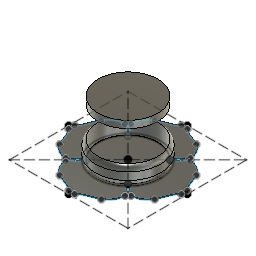
base (Autodesk Fusion 360 design; units mm, degrees)
Autodesk Fusion 360 part; units mm, degrees
note: some values were not read from the file. Set by a fixed rule: which sketch regions a step uses.
sketch "Sketch1" plane through (0, 0, 0) normal (0, 0, 1) x (1, 0, 0)
  line L0 (100, -100) -> (-100, -100) construction
  line L1 (-100, -100) -> (-100, 100) construction
  line L2 (-100, 100) -> (100, 100) construction
  line L3 (100, 100) -> (100, -100) construction
  line L4 (100, -100) -> (-100, 100) construction
  line L5 (-100, -100) -> (100, 100) construction
  circle A0 centre (0, 0) radius 50
  circle A1 centre (0, 0) radius 55
  spline S0 degree 5 poles (35.3553, 35.3553) (35.8403, 36.4134) (36.8629, 38.4351) (38.5545, 41.1842) (41.1261, 44.282) (44.8567, 47.2035) (49.0683, 49.1653) (53.6877, 50.1538) (58.5924, 50.1512) (63.5907, 49.1325) (68.4505, 47.0807) (72.944, 44.008) (76.8867, 39.9747) (80.1793, 35.1099) (82.8485, 29.6311) (85.0884, 23.8652) (87.1733, 18.1914) (89.3708, 12.986) (91.8573, 8.5668) (94.6261, 5.1359) (97.4133, 2.7271) (99.5747, 1.1383) (100.4135, 0) (99.5747, -1.1383) (97.4133, -2.7271) (94.6261, -5.1359) (91.8573, -8.5668) (89.3708, -12.986) (87.1733, -18.1914) (85.0884, -23.8652) (82.8485, -29.6311) (80.1793, -35.1099) (76.8867, -39.9747) (72.944, -44.008) (68.4505, -47.0807) (63.5907, -49.1325) (58.5924, -50.1512) (53.6877, -50.1538) (49.0683, -49.1653) (44.8567, -47.2035) (41.1261, -44.282) (38.5545, -41.1842) (36.8629, -38.4351) (35.8403, -36.4134) (35.3553, -35.3553) knots 0 0 0 0 0 0 0.025 0.05 0.075 0.1 0.125 0.15 0.175 0.2 0.225 0.25 0.275 0.3 0.325 0.35 0.375 0.4 0.425 0.45 0.475 0.5 0.525 0.55 0.575 0.6 0.625 0.65 0.675 0.7 0.725 0.75 0.775 0.8 0.825 0.85 0.875 0.9 0.925 0.95 0.975 1 1 1 1 1 1
  spline S1 degree 5 poles (-35.3553, 35.3553) (-36.4134, 35.8403) (-38.4351, 36.8629) (-41.1842, 38.5545) (-44.282, 41.1261) (-47.2035, 44.8567) (-49.1653, 49.0683) (-50.1538, 53.6877) (-50.1512, 58.5924) (-49.1325, 63.5907) (-47.0807, 68.4505) (-44.008, 72.944) (-39.9747, 76.8867) (-35.1099, 80.1793) (-29.6311, 82.8485) (-23.8652, 85.0884) (-18.1914, 87.1733) (-12.986, 89.3708) (-8.5668, 91.8573) (-5.1359, 94.6261) (-2.7271, 97.4133) (-1.1383, 99.5747) (0, 100.4135) (1.1383, 99.5747) (2.7271, 97.4133) (5.1359, 94.6261) (8.5668, 91.8573) (12.986, 89.3708) (18.1914, 87.1733) (23.8652, 85.0884) (29.6311, 82.8485) (35.1099, 80.1793) (39.9747, 76.8867) (44.008, 72.944) (47.0807, 68.4505) (49.1325, 63.5907) (50.1512, 58.5924) (50.1538, 53.6877) (49.1653, 49.0683) (47.2035, 44.8567) (44.282, 41.1261) (41.1842, 38.5545) (38.4351, 36.8629) (36.4134, 35.8403) (35.3553, 35.3553) knots 0 0 0 0 0 0 0.025 0.05 0.075 0.1 0.125 0.15 0.175 0.2 0.225 0.25 0.275 0.3 0.325 0.35 0.375 0.4 0.425 0.45 0.475 0.5 0.525 0.55 0.575 0.6 0.625 0.65 0.675 0.7 0.725 0.75 0.775 0.8 0.825 0.85 0.875 0.9 0.925 0.95 0.975 1 1 1 1 1 1
  spline S2 degree 5 poles (-35.3553, -35.3553) (-35.8403, -36.4134) (-36.8629, -38.4351) (-38.5545, -41.1842) (-41.1261, -44.282) (-44.8567, -47.2035) (-49.0683, -49.1653) (-53.6877, -50.1538) (-58.5924, -50.1512) (-63.5907, -49.1325) (-68.4505, -47.0807) (-72.944, -44.008) (-76.8867, -39.9747) (-80.1793, -35.1099) (-82.8485, -29.6311) (-85.0884, -23.8652) (-87.1733, -18.1914) (-89.3708, -12.986) (-91.8573, -8.5668) (-94.6261, -5.1359) (-97.4133, -2.7271) (-99.5747, -1.1383) (-100.4135, 0) (-99.5747, 1.1383) (-97.4133, 2.7271) (-94.6261, 5.1359) (-91.8573, 8.5668) (-89.3708, 12.986) (-87.1733, 18.1914) (-85.0884, 23.8652) (-82.8485, 29.6311) (-80.1793, 35.1099) (-76.8867, 39.9747) (-72.944, 44.008) (-68.4505, 47.0807) (-63.5907, 49.1325) (-58.5924, 50.1512) (-53.6877, 50.1538) (-49.0683, 49.1653) (-44.8567, 47.2035) (-41.1261, 44.282) (-38.5545, 41.1842) (-36.8629, 38.4351) (-35.8403, 36.4134) (-35.3553, 35.3553) knots 0 0 0 0 0 0 0.025 0.05 0.075 0.1 0.125 0.15 0.175 0.2 0.225 0.25 0.275 0.3 0.325 0.35 0.375 0.4 0.425 0.45 0.475 0.5 0.525 0.55 0.575 0.6 0.625 0.65 0.675 0.7 0.725 0.75 0.775 0.8 0.825 0.85 0.875 0.9 0.925 0.95 0.975 1 1 1 1 1 1
  spline S3 degree 5 poles (35.3553, -35.3553) (36.4134, -35.8403) (38.4351, -36.8629) (41.1842, -38.5545) (44.282, -41.1261) (47.2035, -44.8567) (49.1653, -49.0683) (50.1538, -53.6877) (50.1512, -58.5924) (49.1325, -63.5907) (47.0807, -68.4505) (44.008, -72.944) (39.9747, -76.8867) (35.1099, -80.1793) (29.6311, -82.8485) (23.8652, -85.0884) (18.1914, -87.1733) (12.986, -89.3708) (8.5668, -91.8573) (5.1359, -94.6261) (2.7271, -97.4133) (1.1383, -99.5747) (0, -100.4135) (-1.1383, -99.5747) (-2.7271, -97.4133) (-5.1359, -94.6261) (-8.5668, -91.8573) (-12.986, -89.3708) (-18.1914, -87.1733) (-23.8652, -85.0884) (-29.6311, -82.8485) (-35.1099, -80.1793) (-39.9747, -76.8867) (-44.008, -72.944) (-47.0807, -68.4505) (-49.1325, -63.5907) (-50.1512, -58.5924) (-50.1538, -53.6877) (-49.1653, -49.0683) (-47.2035, -44.8567) (-44.282, -41.1261) (-41.1842, -38.5545) (-38.4351, -36.8629) (-36.4134, -35.8403) (-35.3553, -35.3553) knots 0 0 0 0 0 0 0.025 0.05 0.075 0.1 0.125 0.15 0.175 0.2 0.225 0.25 0.275 0.3 0.325 0.35 0.375 0.4 0.425 0.45 0.475 0.5 0.525 0.55 0.575 0.6 0.625 0.65 0.675 0.7 0.725 0.75 0.775 0.8 0.825 0.85 0.875 0.9 0.925 0.95 0.975 1 1 1 1 1 1
  point P0 (35.3553, 35.3553)
  point P1 (35.3553, -35.3553)
  point P2 (55, 50)
  point P3 (80, 35)
  point P4 (95, 5)
  point P5 (100, 0)
  point P6 (95, -5)
  point P7 (80, -35)
  point P8 (55, -50)
  point P9 (-50, 55)
  point P10 (-35, 80)
  point P11 (-5, 95)
  point P12 (0, 100)
  point P13 (5, 95)
  point P14 (35, 80)
  point P15 (50, 55)
  point P16 (-55, -50)
  point P17 (-80, -35)
  point P18 (-95, -5)
  point P19 (-100, 0)
  point P20 (-95, 5)
  point P21 (-80, 35)
  point P22 (-55, 50)
  point P23 (50, -55)
  point P24 (35, -80)
  point P25 (5, -95)
  point P26 (0, -100)
  point P27 (-5, -95)
  point P28 (-35, -80)
  point P29 (-50, -55)
  dimension "d1" = 200
  dimension "d2" = 200
  dimension "d3" = 100
  dimension "d4" = 110
  dimension "d15" = 360
  constraint horizontal L0
  constraint perpendicular L0 L1
  constraint parallel L0 L2
  constraint parallel L1 L3
  constraint coincident L4 A0.centre
  constraint coincident L5 A0.centre
  constraint coincident A0.centre A1.centre
  constraint coincident A0 P0
  constraint coincident L5 P0
  constraint coincident A0 P1
  constraint coincident L4 P1
  constraint midpoint L3 P5
  constraint coincident P1 S0.end
  measures "d1" distance of L1.end L2.end
  measures "d2" distance of L0.end L1.end
  measures "d3" diameter of A0
  measures "d4" diameter of A1
extrude "Extrude4" add sketch "Sketch1" along normal blind 1 contours A0 A1 S1 S3 | A0 A1 S0 S2 | A0 A1 S0 S2 | A0 A1 S1 S3 | A1 S0 S1 S2 | A1 S0 S1 S3 | A1 S0 S2 S3 | A1 S1 S2 S3 makes body 1 at (76.9692, 2.241, 1)
extrude "Extrude2" add sketch "Sketch1" along normal blind 1 separate body contours A0 makes body 2
extrude "Extrude1" add sketch "Sketch1" along normal blind 30 separate body contours A0 A1 S1 S3 | A0 A1 S0 S2 | A1 S0 S1 | A0 A1 S0 S2 | A1 S0 S3 | A0 A1 S1 S3 | A1 S1 S2 | A1 S2 S3 picked at (36.5447, 36.5447) picked at (36.5447, -36.5447) picked at (-36.5447, 36.5447) picked at (-36.5447, -36.5447) makes body 3
fillet "Fillet1" radius 10 1 faces at (54.7267, -5.4762, 20) on bodies 3
extrude "Extrude3" add 1 faces at (-19.2634, 8.9959, 1) along direction (0, 0, 1) blind 12 from surface at 80 separate body on bodies 2 makes body 4
